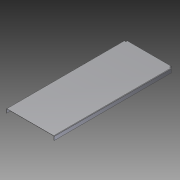
# Autodesk Inventor part: Cart Base
Saved by Autodesk Inventor 2012 (Build 160160000, 160)
## iProperties
Created: 2011-10-13
Part Number: Cart Base
Material: Default
Document SubType Name: Sheet Metal
Designer: Tushar
Density: 1 g/cm^3
Sheet Metal Rule: Default
Author: Tushar
Autodesk Inventor part; units mm, degrees
ref_plane "YZ Plane" through (0, 0, 0) normal (1, 0, 0) x (0, 1, 0)
ref_plane "XZ Plane" through (0, 0, 0) normal (0, 1, 0) x (-1, 0, 0)
ref_plane "XY Plane" through (0, 0, 0) normal (0, 0, 1) x (1, 0, 0)
sketch "Sketch2" plane through (0, 0, 0) normal (0, 1, 0) x (-1, 0, 0)
  line L0 (-304.8, -762) -> (304.8, -762)
  line L1 (304.8, -762) -> (304.8, 762)
  line L2 (304.8, 762) -> (-304.8, 762)
  line L3 (-304.8, 762) -> (-304.8, -762)
  line L4 (304.8, -762) -> (279.4, -762)
  line L5 (279.4, -762) -> (279.4, -736.6)
  line L6 (279.4, -736.6) -> (304.8, -736.6)
  line L7 (304.8, -736.6) -> (304.8, -762)
  line L8 (-304.8, -762) -> (-279.4, -762)
  line L9 (-279.4, -762) -> (-279.4, -736.6)
  line L10 (-279.4, -736.6) -> (-304.8, -736.6)
  line L11 (-304.8, -736.6) -> (-304.8, -762)
  point P0 (0, 0)
  dimension "d0" = 304.8
  dimension "d1" = 304.8
  dimension "d2" = 762
  dimension "d3" = 762
  dimension "d4" = 25.4
  dimension "d5" = 25.4
  dimension "d6" = 25.4
  dimension "d7" = 25.4
  measures "d0" distance from line of L1 point (0, 0)
  measures "d1" distance from line of L3 point (0, 0)
  measures "d2" distance from line of L2 point (0, 0)
  measures "d3" distance from line of L0 point (0, 0)
  measures "d4" distance of L5.end L6.end
  measures "d5" distance of L4.end L5.end
  measures "d6" distance of L10.end L9.end
  measures "d7" distance of L8.end L9.end
extrude "Plate1" add sketch "Sketch2" against normal blind 3.048 contours L9 L10 L3 L2 L1 L6 L5 L0
sketch "Sketch3" plane through (-301.752, 0, -736.6) normal (-1, 0, 0) x (0, -1, 0)
  line L0 (0, 1498.6) -> (0, 0)
  line L1 (0, 0) -> (50.8, 0)
  line L2 (50.8, 0) -> (50.8, 1498.6)
  line L3 (50.8, 1498.6) -> (0, 1498.6)
  constraints: 4 end point, 4 other
edge flange "Flange1" height 50.8 angle 90 thickness 3.048 bend radius 3.048 thickness toward (-1, 0, 0) relief straight relief width 3.048 relief depth 1.524 corner gap 3.048 corner form 0 edges at (-304.8, -3.048, 12.7) (304.8, -3.048, 12.7) (0, -3.048, -762) wall of the first edge with corners at (-301.752, 0, 762) (-301.752, 0, -736.6) (-301.752, -50.8, -736.6) (-301.752, -50.8, 762)
bend "Bend1"
corner "Corner1"
equation "\"d9\" = BendReliefWidth"
equation "\"d10\" = BendReliefDepth"
equation "\"d11\" = MinimumRemnant"
equation "\"d12\" = BendRadius"
equation "\"d15\" = BendRadius"
equation "\"d16\" = CornerReliefSize"
equation "\"d17\" = GapSize"
equation "\"d18\" = JacobiRadiusSize"
equation "\"d1\" = d0"
equation "\"d3\" = d2"
equation "\"BendRadius\" = Thickness"
equation "\"BendReliefWidth\" = Thickness"
equation "\"BendReliefDepth\" = 0.5 * Thickness"
equation "\"CornerReliefSize\" = 4 * Thickness"
equation "\"MinimumRemnant\" = 2 * Thickness"
equation "\"TransitionRadius\" = BendRadius"
equation "\"JacobiRadiusSize\" = BendRadius"
equation "\"GapSize\" = Thickness"
equation "\"d8\" = BendRadius"
equation "\"Thickness\" = 3.048"
body "Solid1"
